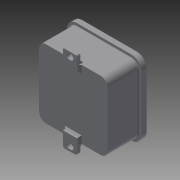
# Autodesk Inventor part: power_conduit_box
Saved by Autodesk Inventor 2013 SP2 (Build 170200200, 200)
## iProperties
Created: 2018-10-25
Part Number: power_conduit_box
Material: Generic
Document SubType Name: Modeling
Designer: alex
Density: 1 g/cm^3
Mass: 180.864 g
Surface Area: 216.286 cm^2
Volume: 180.864 cm^3
Author: alex
Autodesk Inventor part; units mm, degrees
ref_plane "YZ Plane" through (0, 0, 0) normal (1, 0, 0) x (0, 1, 0)
sketch "Sketch1" plane through (0, 0, 0) normal (0, 1, 0) x (-1, 0, 0)
  line L0 (36.4723, -39.8734) -> (-32.5277, -39.8734)
  line L1 (-32.5277, -39.8734) -> (-32.5277, 29.1266)
  line L2 (-32.5277, 29.1266) -> (36.4723, 29.1266)
  line L3 (36.4723, 29.1266) -> (36.4723, -39.8734)
  line L4 (36.4723, -39.8734) -> (-32.5277, 29.1266) construction
  line L5 (-32.5277, -39.8734) -> (36.4723, 29.1266) construction
  point P0 (0, 0)
  point P1 (1.9723, -5.3734)
  dimension "d0" = 69
  dimension "d1" = 69
  constraints: 12 end point, 2 midpoint, 2 parallel, 1 horizontal, 1 perpendicular
  measures "d0" distance of L1.end L2.end
  measures "d1" distance of L0.end L1.end
extrude "Extrusion1" add sketch "Sketch1" along normal blind 31
fillet "Fillet1" radius 7 4 edges at (32.5277, 15.5, 29.1266) (-36.4723, 15.5, 29.1266) (-36.4723, 15.5, -39.8734) (32.5277, 15.5, -39.8734)
sketch "Sketch2" plane through (0, 31, 0) normal (0, 1, 0) x (1, 0, 0)
  arc A0 (32.5277, 32.8734) -> (25.5277, 39.8734) centre (25.5277, 32.8734) ccw projected
  line L0 (25.5277, 39.8734) -> (-29.4723, 39.8734) projected
  arc A1 (-29.4723, 39.8734) -> (-36.4723, 32.8734) centre (-29.4723, 32.8734) ccw projected
  line L1 (-36.4723, 32.8734) -> (-36.4723, -22.1266) projected
  arc A2 (-36.4723, -22.1266) -> (-29.4723, -29.1266) centre (-29.4723, -22.1266) ccw projected
  line L2 (-29.4723, -29.1266) -> (25.5277, -29.1266) projected
  arc A3 (25.5277, -29.1266) -> (32.5277, -22.1266) centre (25.5277, -22.1266) ccw projected
  line L3 (32.5277, -22.1266) -> (32.5277, 32.8734) projected
  line L4 (-29.4723, 42.8734) -> (25.5277, 42.8734)
  arc A4 (35.5277, 32.8734) -> (25.5277, 42.8734) centre (25.5277, 32.8734) ccw
  line L5 (35.5277, 32.8734) -> (35.5277, -22.1266)
  arc A5 (25.5277, -32.1266) -> (35.5277, -22.1266) centre (25.5277, -22.1266) ccw
  line L6 (25.5277, -32.1266) -> (-29.4723, -32.1266)
  arc A6 (-39.4723, -22.1266) -> (-29.4723, -32.1266) centre (-29.4723, -22.1266) ccw
  line L7 (-39.4723, -22.1266) -> (-39.4723, 32.8734)
  arc A7 (-29.4723, 42.8734) -> (-39.4723, 32.8734) centre (-29.4723, 32.8734) ccw
  point P0 (0, 0)
  dimension "d5" = 3
  constraints: 8 end point, 8 point on circle, 4 centre point, 7 other
  measures "d5" distance between parallel lines of L0 L4
extrude "Extrusion2" add sketch "Sketch2" along normal blind 6 contours L3 A3 L2 A2 L1 A1 L0 A0 | L4 A4 L5 A5 L6 A6 L7 A7
fillet "Fillet2" radius 1 8 edges at (-1.9723, 31, 29.1266) (-34.422, 31, 27.0763) (-36.4723, 31, -5.3734) (-34.422, 31, -37.8232) (-1.9723, 31, -39.8734) (30.4775, 31, -37.8232) (32.5277, 31, -5.3734) (30.4775, 31, 27.0763)
fillet "Fillet3" radius 1 8 edges at (32.5988, 37, 29.1977) (35.5277, 37, -5.3734) (32.5988, 37, -39.9445) (-1.9723, 37, -42.8734) (-36.5433, 37, -39.9445) (-39.4723, 37, -5.3734) (-36.5433, 37, 29.1977) (-1.9723, 37, 32.1266)
sketch "Sketch3" plane through (0, 0, 0) normal (0, -1, 0) x (1, 0, 0)
  line L0 (32.5277, -32.8734) -> (32.5277, 22.1266) projected
  line L1 (25.5277, 29.1266) -> (-29.4723, 29.1266) projected
  line L2 (-36.4723, 22.1266) -> (-36.4723, -32.8734) projected
  line L3 (-8.9723, 38.1266) -> (5.0277, 38.1266)
  line L4 (5.0277, 38.1266) -> (5.0277, 23.1266)
  line L5 (5.0277, 23.1266) -> (-8.9723, 23.1266)
  line L6 (-8.9723, 23.1266) -> (-8.9723, 38.1266)
  line L7 (-8.9723, 23.1266) -> (-36.4723, 23.1266)
  line L8 (5.0277, 23.1266) -> (32.5277, 23.1266)
  point P0 (0, 0)
  dimension "d10" = 14
  dimension "d12" = 15
  dimension "d13" = 9
  constraints: 12 end point, 3 perpendicular, 2 parallel, 2 point on line, 1 collinear, 1 horizontal
  measures "d10" distance of L4.end L5.end
  measures "d12" distance of L5.end L3.start
  measures "d13" distance between parallel lines of L3 L1
extrude "Extrusion3" add sketch "Sketch3" along normal blind 3.5
chamfer "Chamfer1" distance 1.5 angle 45 3 edges at (-8.9723, 0, 26.1266) (-1.9723, 0, 23.1266) (5.0277, 0, 26.1266)
sketch "Sketch4" plane through (0, 0, 0) normal (0, 1, 0) x (1, 0, 0)
  line L0 (5.0277, -29.1266) -> (-8.9723, -29.1266) projected
  line L1 (-8.9723, -38.1266) -> (5.0277, -38.1266) projected
  line L2 (-1.9723, -38.1266) -> (-1.9723, -29.1266)
  line L3 (-1.9723, -33.6266) -> (-0.9723, -33.6266)
  line L4 (-1.9723, -33.6266) -> (-2.9723, -33.6266)
  circle A0 centre (-2.9723, -33.6266) radius 2.5
  circle A1 centre (-0.9723, -33.6266) radius 2.5
  line L5 (-2.9723, -31.1266) -> (-0.9723, -31.1266)
  line L6 (-0.9723, -31.1266) -> (-0.9723, -36.1266)
  line L7 (-0.9723, -36.1266) -> (-2.9723, -36.1266)
  line L8 (-2.9723, -36.1266) -> (-2.9723, -31.1266)
  point P0 (0, 0)
  dimension "d21" = 5
  dimension "d22" = 5
  dimension "d19" = 1
  dimension "d20" = 1
  constraints: 14 end point, 3 equal length, 3 midpoint, 2 coincident, 2 perpendicular, 2 vertical alignment, 1 horizontal, 4 other
  measures "d19" distance of L3.start L3.end
  measures "d20" distance of L3.start L4.end
extrude "Extrusion4" cut sketch "Sketch4" against normal blind 3.5
sketch "Sketch5" plane through (5.0277, 0, 38.1266) normal (1, 0, 0) x (0, 0, -1)
  line L0 (0, 0) -> (9, 0) projected
  line L1 (9, 0) -> (9, 30) projected
  line L2 (9, -1.5) -> (9, 0) projected
  line L3 (9, 0) -> (9, -1.5) projected
  line L4 (9, -1.5) -> (9, 0) projected
  line L5 (9, -1.5) -> (9, 0) projected
  line L6 (9, 30) -> (9, 0) projected
  line L7 (6, 0) -> (9, 3)
  line L8 (6, 0) -> (10.2426, 0) construction
  line L9 (6, 0) -> (9, 0)
  line L10 (9, 3) -> (9, 0)
  point P0 (38.1266, 0)
  dimension "d25" = 45
  dimension "d26" = 3
  constraints: 8 end point, 2 collinear, 2 point on line, 1 equal length, 1 horizontal
  measures "d25" angle of L8 L7
  measures "d26" distance of L0.end L7.start
extrude "Extrusion5" add sketch "Sketch5" against normal blind 1.5
ref_plane "Work Plane1" through (-1.9723, -3.5, 38.1266) normal (1, 0, 0) x (0, 0, -1)
mirror "Mirror1" about plane through (-1.9723, -3.5, 38.1266) normal (1, 0, 0) of "Extrusion5"
fillet "Fillet4" radius 1.5 2 edges at (-8.9723, -1.75, 38.1266) (5.0277, -1.75, 38.1266)
ref_plane "Work Plane2" through (-29.4723, 30, -5.3734) normal (0, 0, 1) x (1, 0, 0)
mirror "Mirror2" about plane through (-29.4723, 30, -5.3734) normal (0, 0, 1) of "Extrusion3", "Chamfer1", "Extrusion4", "Extrusion5", "Mirror1", "Fillet4"
ref_plane "Work Plane3" through (-1.9723, -3.5, -48.8734) normal (-1, 0, 0) x (0, 0, 1)
body "Solid1"
